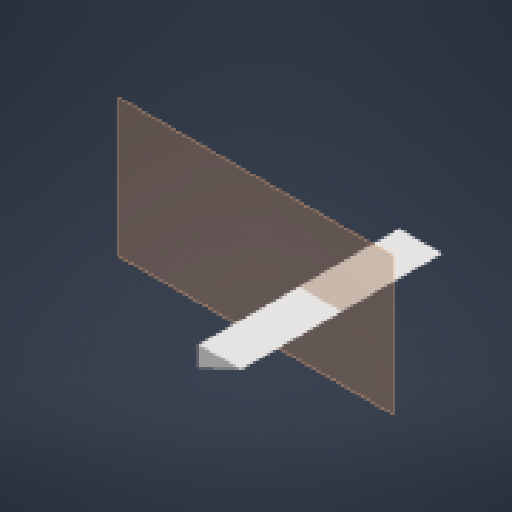
# Autodesk Inventor part: main body blade part
Saved by Autodesk Inventor 2026.2 (Build 302298010, 298A)
## iProperties
Created: 2026-04-08
Part Number: main body blade part
Material: Generic
Document SubType Name: Modeling
Designer: Martin
Density: 1 g/cm^3
Appearance: Default
Author: Martin
Autodesk Inventor part; units mm, degrees
ref_plane "YZ Plane" through (0, 0, 0) normal (1, 0, 0) x (0, 1, 0)
ref_plane "XZ Plane" through (0, 0, 0) normal (0, 1, 0) x (-1, 0, 0)
ref_plane "XY Plane" through (0, 0, 0) normal (0, 0, 1) x (1, 0, 0)
ref_plane "Work Plane1" through (0, 0, 0) normal (0, 0, 1) x (1, 0, 0)
sketch "Sketch1" plane through (0, 0, 0) normal (0, 0, 1) x (1, 0, 0)
  line L0 (92.4014, -2) -> (71.0429, -11.9596) projected
  line L1 (71.0429, -11.9596) -> (72.3108, -14.6785) projected
  line L2 (72.3108, -14.6785) -> (99.5, -2) projected
  line L3 (99.5, -2) -> (92.4014, -2) projected
  line L4 (79.5612, -11.2976) -> (78.5047, -9.0318)
  line L5 (82.2802, -10.0297) -> (81.2236, -7.764)
  line L6 (81.4655, -7.0995) -> (81.2236, -7.764)
  line L7 (77.8402, -8.79) -> (78.5047, -9.0318)
  line L8 (92.4014, -2) -> (71.0429, -2)
  line L9 (71.0429, -2) -> (71.0429, -11.9596)
  line L10 (71.0429, -11.9596) -> (53.5429, -42.2705)
  line L11 (53.5429, -42.2705) -> (52.2439, -41.5205)
  line L12 (52.6769, -40.7705) -> (69.7439, -11.2096)
  line L13 (69.7439, -11.2096) -> (71.0429, -11.9596)
  line L14 (71.0429, -11.9596) -> (106.0429, -11.9596) construction
  line L15 (53.5429, -42.2705) -> (42.5429, -42.2705)
  line L16 (42.5429, -42.2705) -> (42.5429, -40.7705)
  line L17 (42.5429, -40.7705) -> (52.6769, -40.7705)
  point P0 (0, 0)
  dimension "d0" = 35
  dimension "d1" = 120
  dimension "d2" = 1.5
  dimension "d3" = 11
  dimension "d4" = 1.5
  constraints: 28 end point, 4 perpendicular, 3 horizontal, 2 parallel, 1 equal length, 10 other
  measures "d0" distance of L0.end L10.end
  measures "d1" angle of L10 L14
  measures "d2" distance of L10.end L11.end
  measures "d3" distance of L10.end L15.end
  measures "d4" distance of L15.end L16.end
extrude "Extrusion1" add sketch "Sketch1" along normal mid plane 99.5 contours L0 L9 L8
